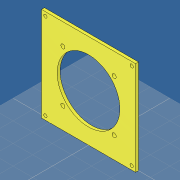
# Autodesk Inventor part: DayLightGlow_SpeakerBase
Saved by Autodesk Inventor 2019 (Build 230136000, 136)
## iProperties
Created: 2019-01-03
Part Number: DayLightGlow_SpeakerBase
Material: Generisch
Document SubType Name: Modeling
Designer: Stefan
Mass: 17.7218 g
Surface Area: 138.562 cm^2
Volume: 17.7218 cm^3
Density: 1 g/cm^3
Appearance: Glatt - Gelb
Author: Stefan
Autodesk Inventor part; units mm, degrees
ref_plane "YZ Plane" through (0, 0, 0) normal (1, 0, 0) x (0, 1, 0)
ref_plane "XZ Plane" through (0, 0, 0) normal (0, 1, 0) x (-1, 0, 0)
ref_plane "XY Plane" through (0, 0, 0) normal (0, 0, 1) x (1, 0, 0)
sketch "Skizze1" plane through (0, 0, 0) normal (0, 0, 1) x (1, 0, 0)
  line L0 (48, -48) -> (-48, -48)
  line L1 (-48, -48) -> (-48, 48)
  line L2 (-48, 48) -> (48, 48)
  line L3 (48, 48) -> (48, -48)
  line L4 (48, -48) -> (-48, 48) construction
  line L5 (-48, -48) -> (48, 48) construction
  circle A0 centre (0, 0) radius 32
  circle A1 centre (0, 0) radius 37 construction
  line L6 (-40, 40) -> (-48, 40)
  line L7 (-48, 40) -> (-48, 48)
  line L8 (-48, 48) -> (-40, 48)
  line L9 (-40, 48) -> (-40, 40)
  line L10 (-40, 40) -> (-48, 48) construction
  line L11 (-48, 40) -> (-40, 48) construction
  line L12 (-40, -40) -> (-48, -40)
  line L13 (-48, -40) -> (-48, -48)
  line L14 (-48, -48) -> (-40, -48)
  line L15 (-40, -48) -> (-40, -40)
  line L16 (-40, -40) -> (-48, -48) construction
  line L17 (-48, -40) -> (-40, -48) construction
  line L18 (40, -40) -> (48, -40)
  line L19 (48, -40) -> (48, -48)
  line L20 (48, -48) -> (40, -48)
  line L21 (40, -48) -> (40, -40)
  line L22 (40, -40) -> (48, -48) construction
  line L23 (48, -40) -> (40, -48) construction
  line L24 (40, 40) -> (48, 40)
  line L25 (48, 40) -> (48, 48)
  line L26 (48, 48) -> (40, 48)
  line L27 (40, 48) -> (40, 40)
  line L28 (40, 40) -> (48, 48) construction
  line L29 (48, 40) -> (40, 48) construction
  point P0 (-26.163, 26.163)
  point P1 (26.163, 26.163)
  point P2 (26.163, -26.163)
  point P3 (-26.163, -26.163)
  point P4 (-44, 44)
  point P5 (-44, -44)
  point P6 (44, -44)
  point P7 (44, 44)
  point P8 (-44, 44)
  point P9 (44, 44)
  point P10 (-44, -44)
  point P11 (44, -44)
  dimension "d0" = 96
  dimension "d1" = 96
  dimension "d41" = 64
  dimension "d42" = 74
  dimension "d43" = 8
  dimension "d44" = 8
  constraints: 60 end point, 10 midpoint, 10 parallel, 6 coincident, 6 equal length, 5 horizontal, 5 perpendicular, 4 point on circle, 4 point on line, 2 centre point
  measures "d0" distance between parallel lines of L0 L2
  measures "d1" distance between parallel lines of L3 L1
  measures "d41" diameter of A0
  measures "d42" diameter of A1
  measures "d43" distance of L8.end L6.start
  measures "d44" distance of L6.start L6.end
extrude "Extrusion1" add sketch "Skizze1" along normal blind 3
hole "Bohrung2" at (-44, 44, 0) at (44, 44, 0) at (-44, -44, 0) at (44, -44, 0) direction (0, 0, 1) diameter 3.4 end through all
hole "Bohrung3" at (-26.163, 26.163, 0) at (26.163, 26.163, 0) at (26.163, -26.163, 0) at (-26.163, -26.163, 0) direction (0, 0, 1) diameter 4.2 end through all
equation "\"d0\" = d1"
